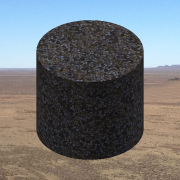
# Autodesk Inventor part: 2p3cem
Saved by Autodesk Inventor 2013 SP2 (Build 170200200, 200)
## iProperties
Company: HERA Project
Created: 2013-06-11
Part Number: 2p3cem
Material: Concrete
Document SubType Name: Modeling
Designer: David DeBoer
Density: 2.40731 g/cm^3
Description: Support stand cement
Mass: 39212.8 g
Surface Area: 3562.79 cm^2
Volume: 16289.1 cm^3
Author: David DeBoer
Title: Support stand cement
Autodesk Inventor part; units mm, degrees
ref_plane "YZ Plane" through (0, 0, 0) normal (1, 0, 0) x (0, 1, 0)
ref_plane "XZ Plane" through (0, 0, 0) normal (0, 1, 0) x (-1, 0, 0)
ref_plane "XY Plane" through (0, 0, 0) normal (0, 0, 1) x (1, 0, 0)
sketch "Sketch1" plane through (0, 0, 0) normal (0, 1, 0) x (-1, 0, 0)
  circle A0 centre (0, 0) radius 142.875
  dimension "d0" = 285.75
  constraints: 1 centre point, 1 coincident
  measures "d0" diameter of A0
extrude "Extrusion1" add sketch "Sketch1" against normal blind 254
body "Solid1"
